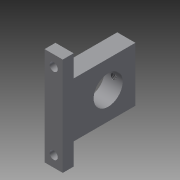
# Autodesk Inventor part: SHTA16-25_b
Saved by Autodesk Inventor 2014 SP2 (Build 180246200, 246)
## iProperties
Created: 2019-04-24
Part Number: SHTA16-25_b
Material: Generic
Catalog Web Link: www.cadenas.de
Description: SHTB, SHTM, SHTS, SHTA_body-Shaft Supports - T-Shaped Set Screw (Machined) - Standard - w/o Dowel Hole - Height H Selectable Type
Vendor: MISUMI
Document SubType Name: Modeling
Designer: psadmin
Manufacturer: MISUMI
Mass: 11.1796 g
Surface Area: 48.2799 cm^2
Volume: 11.1796 cm^3
Density: 1 g/cm^3
Appearance: PSOLRGB-192-192-192
Category: PARTsolutions
Company: MISUMI
Title: SHTA16-25
Author: Cadenas PARTsolutions
Comments: Shaft Supports - T-Shaped Set Screw (Machined) - Standard - w/o Dowel Hole - Height H Selectable Type
PSOL_IDENT_0: {$CADENAS_DATA\23d-libs\misumi\metric\02_shaft_supports\shtb\shtb_b.prj},191 {VTYP=3D},{NB=SHTA16-25
PSOL_IDENT_1: _b},{LINA=SHTA16-25},{NN=SHTB, SHTM, SHTS, SHTA_body},{DATE=30.03.2018 01:12:49},{GEOMDATE=19.11.201
PSOL_IDENT_2: 5 01:06:00},{VERSION=},{LINEID=100},{WBVAR=MAT,ST,H},{WBNUMERIC=H}  {NB=SHTA16-25_b},{LINA=SHTA16-25
PSOL_IDENT_3: },{KT=DUMMY},{PN=SHTA16-25},{TYPE=SHTA},{MAT=A6063},{ST=CA},{STALG='CA','Clear Anodize'},{D=16},{H=2
PSOL_IDENT_4: 5},{HALG=15,20,25,30,40},{L=54},{H1=40},{T=10},{S=6},{W=30},{M=M4},{L1=42},{DD=4.5},{THMD=4},{HM=6.0
PSOL_IDENT_5: 00},{H0=15},{HH=15,20,25,30,40}
NN: SHTB, SHTM, SHTS, SHTA_body
NT: Shaft Supports - T-Shaped Set Screw (Machined) - Standard - w/o Dowel Hole - Height H Selectable Type
NB: SHTA16-25_b
NBSYN: $PN._b
LINA: SHTA16-25
PN: SHTA16-25
MAT: 6063 Aluminum Alloy
ST: Clear Anodize
D: 16
H: 25
L: 54
H1: 40
T: 10
S: 6
W: 30
M: M4
L1: 42
DD: 4.5
SUPPLIER: MISUMI
ARTICLENO: SHTA16-25_b
BOMINFO: SHTA16-25
CREATOR: CADENAS GmbH
Autodesk Inventor part; units mm, degrees
ref_plane "YZ Plane" through (0, 0, 0) normal (1, 0, 0) x (0, 1, 0)
ref_plane "XZ Plane" through (0, 0, 0) normal (0, 1, 0) x (-1, 0, 0)
ref_plane "XY Plane" through (0, 0, 0) normal (0, 0, 1) x (1, 0, 0)
sketch "Sketch_1" plane through (0, 0, 0) normal (1, 0, 0) x (0, 1, 0)
  line L0 (6, 27) -> (0, 27)
  line L1 (0, 27) -> (0, -27)
  line L2 (0, -27) -> (6, -27)
  line L3 (6, -27) -> (6, -15)
  line L4 (6, -15) -> (40, -15)
  line L5 (40, -15) -> (40, 15)
  line L6 (40, 15) -> (6, 15)
  line L7 (6, 15) -> (6, 27)
  constraints: 16 end point
extrude "Extrusion1" add sketch "Sketch_1" along normal mid plane 10
sketch "Sketch2" plane through (-5, 40, 15) normal (0, 1, 0) x (1, 0, 0)
  point P0 (5, 15)
hole "Hole1" at (0, 40, 0) direction (0, -1, 0) diameter 3.242 depth 14.0641 tip angle 120 countersink diameter 4 countersink angle 90 thread size "M4x0.7" class "6H" standard "ISO Metric profile"
sketch "Sketch3" plane through (-5, 0, -27) normal (0, -1, 0) x (1, 0, 0)
  point P0 (5, 6)
hole "Hole2" at (0, 0, -21) direction (0, 1, 0) diameter 4.5 depth 6
pattern_linear "Rectangular Pattern1" count 2 spacing 42 along (0, 0, 1) of "Hole2"
sketch "Sketch4" plane through (5, 0, 0) normal (1, 0, 0) x (0, 0, -1)
  point P0 (0, 25)
hole "Hole3" at (5, 25, 0) direction (-1, 0, 0) diameter 16 depth 10
ref_plane "b_s_XY" through (0, 33, 0) normal (0, 1, 0) x (1, 0, 0)
ref_plane "b_s_YZ" through (0, 33, 0) normal (1, 0, 0) x (0, 0, -1)
ref_plane "b_s_ZX" through (0, 33, 0) normal (0, 0, -1) x (0, 1, 0)
body "Solid1"
